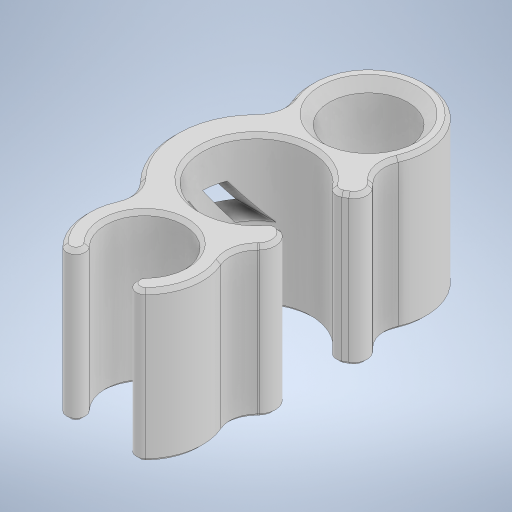
# Autodesk Inventor part: umbilicalClip
Saved by Autodesk Inventor 2024.2 (Build 282272000, 272)
## iProperties
Created: 2024-07-26
Part Number: umbilicalClip
Material: Generic
Document SubType Name: Modeling
Designer: Eric
Density: 1 g/cm^3
Appearance: Default
Author: Eric
Autodesk Inventor part; units mm, degrees
ref_plane "XZ Plane" through (0, 0, 0) normal (0, 1, 0) x (-1, 0, 0)
ref_plane "XY Plane" through (0, 0, 0) normal (0, 0, 1) x (1, 0, 0)
sketch "Sketch1" plane through (0, 0, 0) normal (0, 1, 0) x (-1, 0, 0)
  circle A0 centre (0, 0) radius 2.9
  circle A1 centre (0, -6) radius 2.1
  circle A2 centre (0, 6) radius 2.1
  circle A3 centre (0, 0) radius 4.4
  circle A4 centre (0, -6) radius 3.1
  circle A5 centre (0, 6) radius 3.1
  line L0 (-2.5397, -1.4) -> (-3.8533, -2.1241)
  line L1 (-2.5397, 1.4) -> (-3.8533, 2.1241)
  line L2 (1.2, 7.7234) -> (1.7714, 8.544)
  line L3 (-1.2, 7.7234) -> (-1.7714, 8.544)
  point P0 (-2.1966, -3.8125)
  point P1 (2.1966, -3.8125)
  point P2 (2.1966, 3.8125)
  point P3 (-2.1966, 3.8125)
  dimension "d0" = 5.8
  dimension "d1" = 4.2
  dimension "d2" = 4.2
  dimension "d3" = 6
  dimension "d4" = 6
  dimension "d5" = 1.5
  dimension "d6" = 1
  dimension "d7" = 1
  dimension "d10" = 2.8
  dimension "d11" = 1.4
  dimension "d13" = 2.4
  dimension "d14" = 1.2
  constraints: 8 end point, 8 point on circle, 6 centre point, 4 line through centre, 2 vertical alignment, 1 coincident
  measures "d0" diameter of A0
  measures "d1" diameter of A1
  measures "d2" diameter of A2
  measures "d3" distance of A1.centre point (0, 0)
  measures "d4" distance of A2.centre point (0, 0)
  measures "d5" radial gap between concentric circles of A0 A3
  measures "d6" radial gap between concentric circles of A1 A4
  measures "d7" radial gap between concentric circles of A2 A5
  measures "d10" distance of L1.start L0.start
  measures "d11" vertical distance of point (0, 0) L0.start
  measures "d13" distance of L3.start L2.start
  measures "d14" horizontal distance of A2.centre L2.start
extrude "Extrusion1" add sketch "Sketch1" along normal blind 8 contours L1 A3 A5 A0 | A0 A4 A3 L0 | A5 A3 A4 A0 | A5 A3 A2 | A4 A3 A1 | A5 L3 A2 A3 | A3 A2 L2 A5 | A4 A3 A1
fillet "Fillet1" radius 1.5 4 edges at (2.1966, 4, -3.8125) (-2.1966, 4, -3.8125) (-2.1966, 4, 3.8125) (2.1966, 4, 3.8125)
fillet "Fillet2" radius 0.9 1 edges at (3.8533, 4, 2.1241)
fillet "Fillet3" radius 0.5 2 edges at (2.5397, 4, -1.4) (2.5397, 4, 1.4)
fillet "Fillet4" radius 0.7 1 edges at (3.8533, 4, -2.1241)
fillet "Fillet5" radius 0.5 4 edges at (-1.2, 4, 7.7234) (1.2, 4, 7.7234) (-1.7714, 4, 8.544) (1.7714, 4, 8.544)
ref_plane "Work Plane1" through (-4.4, 0, 0) normal (1, 0, 0) x (0, 1, 0)
sketch "Sketch2" plane through (-4.4, 0, 0) normal (1, 0, 0) x (0, 1, 0)
  line L0 (6, -1.0996) -> (6, 0.0004)
  line L1 (6, 0.0004) -> (4, -1.4)
  line L2 (4, -1.4) -> (4, -2.5)
  line L3 (4, -2.5) -> (6, -1.0996)
  line L4 (6, 0.8504) -> (6, 1.9504)
  line L5 (6, 1.9504) -> (2, -0.8504)
  line L6 (2, -0.8504) -> (2, -1.9504)
  line L7 (2, -1.9504) -> (6, 0.8504)
  line L8 (4, 1.4) -> (4, 2.5)
  line L9 (4, 2.5) -> (2, 1.0996)
  line L10 (2, 1.0996) -> (2, -0.0004)
  line L11 (2, -0.0004) -> (4, 1.4)
  line L12 (2, -0.8504) -> (2, -0.0004) construction
  line L13 (6, 0.0004) -> (6, 0.8504) construction
  line L14 (0, -3.0856) -> (0, 3.0856) construction
  point P0 (0, 0)
  point P1 (0, 0)
  point P2 (0, 0)
  dimension "d19" = 125
  dimension "d20" = 4
  dimension "d21" = 5
  dimension "d22" = 0.85
  dimension "d23" = 2.5
  dimension "d24" = 2
  constraints: 28 end point, 9 parallel, 4 equal length, 4 vertical, 3 collinear, 2 midpoint
  measures "d19" angle of L3 L0
  measures "d20" distance between parallel lines of L4 L10
  measures "d21" distance of L2.end L8.end
  measures "d22" distance of L0.end L4.start
  measures "d23" vertical distance of point (0, 0) L2.end
  measures "d24" horizontal distance of point (0, 0) L9.end
extrude "Extrusion2" cut sketch "Sketch2" along normal up to surface round surface about axis through (0, 0, 0) along (0, 1, 0) radius 2.9 far side no
chamfer "Chamfer1" distance 0.5 angle 45 2 edges at (2.1, 8, -6) (2.1, 0, -6)
chamfer "Chamfer2" distance 0.2 angle 45 48 edges at (-2.9, 8, 0) (2.6007, 8, -1.5722) (3.0635, 8, -1.6887) (3.5317, 8, -2.2372) (3.2621, 8, -2.9527) (2.7304, 8, -3.8687) (0, 8, -9.1) (-2.7304, 8, -3.8687) (-4.4, 8, 0) (-2.7304, 8, 3.8687) (-3.0521, 8, 6.5431) (-1.8281, 8, 8.3066) (-1.458, 8, 8.0939) (-1.3699, 8, 7.768) (0, 8, 3.9) (1.3699, 8, 7.768) (1.458, 8, 8.0939) (1.8281, 8, 8.3066) (3.0521, 8, 6.5431) (2.7304, 8, 3.8687) (3.1572, 8, 3.0646) (3.4173, 8, 2.2851) (2.9536, 8, 1.6282) (2.6007, 8, 1.5722) (-3.0521, 0, 6.5431) (-1.8281, 0, 8.3066) (-1.458, 0, 8.0939) (-1.3699, 0, 7.768) (0, 0, 3.9) (1.3699, 0, 7.768) (1.458, 0, 8.0939) (1.8281, 0, 8.3066) (3.0521, 0, 6.5431) (2.7304, 0, 3.8687) (3.1572, 0, 3.0646) (3.4173, 0, 2.2851) (2.9536, 0, 1.6282) (2.6007, 0, 1.5722) (-2.9, 0, 0) (2.6007, 0, -1.5722) (3.0635, 0, -1.6887) (3.5317, 0, -2.2372) (3.2621, 0, -2.9527) (2.7304, 0, -3.8687) (0, 0, -9.1) (-2.7304, 0, -3.8687) (-4.4, 0, 0) (-2.7304, 0, 3.8687)
body "Solid1"
